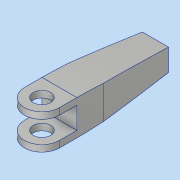
# Autodesk Inventor part: metalClevisis
Saved by Autodesk Inventor 2017 (Build 210142000, 142)
## iProperties
Created: 2016-12-11
Part Number: metalClevisis
Material: Aluminum 6061
Document SubType Name: Modeling
Designer: techn
Density: 2.7 g/cm^3
Appearance: Aluminum - Flat
Author: techn
Autodesk Inventor part; units mm, degrees
ref_plane "YZ Plane" through (0, 0, 0) normal (1, 0, 0) x (0, 1, 0)
ref_plane "XZ Plane" through (0, 0, 0) normal (0, 1, 0) x (-1, 0, 0)
ref_plane "XY Plane" through (0, 0, 0) normal (0, 0, 1) x (1, 0, 0)
sketch "Sketch6" plane through (0, 0, 0) normal (0, 1, 0) x (-1, 0, 0)
  line L0 (0, 0) -> (4, 0)
  line L1 (4, 0) -> (4, -15)
  line L2 (4, -15) -> (0, -15)
  line L3 (0, -15) -> (0, 0)
  dimension "d17" = 4
  dimension "d18" = 15
  constraints: 8 end point, 2 parallel, 1 horizontal, 1 perpendicular
  measures "d17" distance of L1.end L2.end
  measures "d18" distance of L0.end L1.end
extrude "Extrusion5" add sketch "Sketch6" along normal blind 4
sketch "Sketch7" plane through (-4, 0, 0) normal (0, 0, 1) x (1, 0, 0)
  line L0 (0, 0) -> (0, 4) projected
  line L1 (4, 0) -> (4, 4) projected
  line L2 (0, 3.25) -> (4, 3.25)
  line L3 (4, 3.25) -> (4, 0.75)
  line L4 (4, 0.75) -> (0, 0.75)
  line L5 (0, 0.75) -> (0, 3.25)
  line L6 (0, 4) -> (4, 4) projected
  line L7 (4, 0) -> (0, 0) projected
  dimension "d21" = 0.75
  dimension "d22" = 0.75
  constraints: 8 end point, 2 parallel, 2 point on line, 1 horizontal, 1 perpendicular
  measures "d21" distance between parallel lines of L2 L6
  measures "d22" distance between parallel lines of L7 L4
extrude "Extrusion6" cut sketch "Sketch7" against normal blind 4 contours L0 L2 L1 L4
sketch "Sketch8" plane through (0, 4, 0) normal (0, 1, 0) x (1, 0, 0)
  line L0 (-4, 4) -> (0, 4) projected
  line L1 (-4, 15) -> (-4, 0) projected
  line L2 (0, 0) -> (-4, 0) projected
  line L3 (-4, 4) -> (-4, 0)
  circle A0 centre (-2, 2) radius 1
  dimension "d25" = 2
  constraints: 2 end point, 1 centre point, 1 vertical
  measures "d25" diameter of A0
extrude "Extrusion7" cut sketch "Sketch8" against normal blind 4
sketch "Sketch9" plane through (0, 0, -15) normal (0, 0, -1) x (-1, 0, 0)
  line L0 (4, 0) -> (0, 0) projected
  line L1 (4, 0) -> (4, 4) projected
  line L2 (0, 4) -> (4, 4) projected
  line L3 (0, 0) -> (0, 4) projected
  circle A0 centre (2, 2) radius 1
  point P0 (0, 0)
  dimension "d28" = 2
  constraints: 1 centre point
  measures "d28" diameter of A0
extrude "Extrusion8" cut sketch "Sketch9" against normal blind 8 contours A0
sketch "Sketch10" plane through (0, 0, 0) normal (1, 0, 0) x (0, 0, -1)
  line L0 (0, 3.25) -> (4, 3.25) projected
  line L1 (4, 3.25) -> (4, 0.75) projected
  line L2 (4, 0.75) -> (0, 0.75) projected
  line L3 (0, 0) -> (0, 0.75) projected
  line L4 (15, 0) -> (0, 0) projected
  line L5 (15, 0) -> (15, 4) projected
  line L6 (0, 4) -> (15, 4) projected
  line L7 (0, 3.25) -> (0, 4) projected
  line L8 (15, 4) -> (0, 4) projected
  line L9 (4, 4) -> (7.2907, 4) construction
  line L10 (15, 0) -> (15, 4) projected
  line L11 (7.2907, 4) -> (15, 3.25) construction
  spline S0 degree 2 poles (4, 4) (7.2907, 4) (15, 3.25) knots 1 1 1 2 2 2
  line L12 (4, 3.25) -> (4, 0.75) projected
  line L13 (4, 2) -> (3.448, 2)
  line L14 (4, 0) -> (7.2907, 0) construction
  line L15 (7.2907, 0) -> (15, 0.75) construction
  spline S1 degree 2 poles (4, 0) (7.2907, 0) (15, 0.75) knots 1 1 1 2 2 2
  dimension "d31" = 0.75
  constraints: 3 point on line, 3 symmetric about line, 2 end point, 1 horizontal, 1 midpoint, 6 other
  measures "d31" distance of L5.end L11.end
extrude "Extrusion9" cut sketch "Sketch10" against normal blind 8 contours L6 L5 S0
pattern_circular "Circular Pattern1" count 2 over 360 about axis through (-2, 2, -15) along (0, 0, 1) of "Extrusion9"
fillet "Fillet1" radius 2 4 edges at (0, 3.625, 0) (-4, 3.625, 0) (0, 0.375, 0) (-4, 0.375, 0)
chamfer "Chamfer1" distance 8 distance2 0.5 1 edges at (0, 2, -15) measured on face at (0, 2, -14.5)
chamfer "Chamfer2" distance 0.5 distance2 8 1 edges at (-4, 2, -15) measured on face at (-3.5, 2, -15)
body "Solid2"
